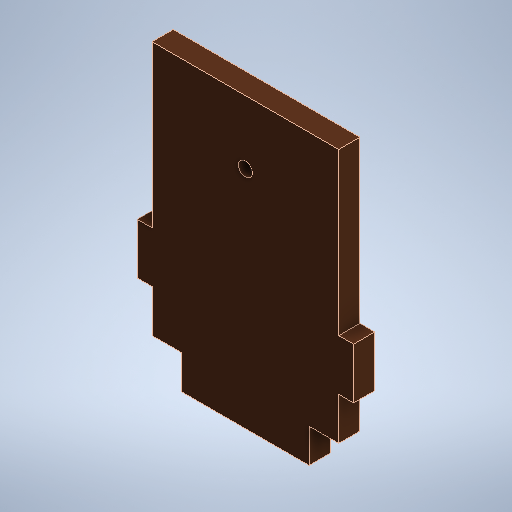
# Autodesk Inventor part: Path Back End
Saved by Autodesk Inventor 2025.4 (Build 294407000, 407)
## iProperties
Created: 2026-04-10
Part Number: Path Back End
Material: Generic
Document SubType Name: Sheet Metal
Designer: lenovo
Density: 1 g/cm^3
Sheet Metal Rule: Default_mm
Appearance: Default(1)
Author: lenovo
Autodesk Inventor part; units mm, degrees
ref_plane "YZ Plane" through (0, 0, 0) normal (1, 0, 0) x (0, 1, 0)
ref_plane "XZ Plane" through (0, 0, 0) normal (0, 1, 0) x (-1, 0, 0)
ref_plane "XY Plane" through (0, 0, 0) normal (0, 0, 1) x (1, 0, 0)
sketch "Sketch1" plane through (0, 0, 0) normal (0, 0, 1) x (1, 0, 0)
  line L0 (-22, -30) -> (22, -30)
  line L1 (22, -30) -> (22, 30)
  line L2 (22, 30) -> (-22, 30)
  line L3 (-22, 30) -> (-22, -30)
  line L4 (-22, -30) -> (22, 30) construction
  line L5 (22, -30) -> (-22, 30) construction
  line L6 (-15, -38) -> (15, -38)
  line L7 (15, -38) -> (15, -30)
  line L8 (15, -30) -> (-15, -30)
  line L9 (-15, -30) -> (-15, -38)
  line L10 (-15, -38) -> (15, -30) construction
  line L11 (15, -38) -> (-15, -30) construction
  circle A0 centre (0, 15) radius 1.65
  point P0 (0, 0)
  point P1 (0, -34)
  point P2 (0, -30)
  point P3 (0, 30)
  dimension "d0" = 44
  dimension "d1" = 60
  dimension "d2" = 30
  dimension "d3" = 8
  dimension "d4" = 3.3
  dimension "d5" = 15
  measures "d0" distance of L1.end L2.end
  measures "d1" distance of L0.end L1.end
  measures "d2" distance of L6.start L6.end
  measures "d3" distance of L6.end L7.end
  measures "d4" diameter of A0
  measures "d5" distance from line of L2 A0.centre
sketch "Sketch2" plane through (0, 0, 5) normal (0, 0, 1) x (1, 0, 0)
  line L0 (22, -30) -> (22, 30)
  line L1 (22, -20) -> (25.5, -20)
  line L2 (25.5, -20) -> (25.5, -8)
  line L3 (25.5, -8) -> (22, -8)
  line L4 (22, -8) -> (22, -20)
  line L5 (22, -30) -> (15, -30)
  line L6 (0, 0) -> (0, -38)
  line L7 (-15, -38) -> (15, -38)
  line L8 (-22, -20) -> (-25.5, -20)
  line L9 (-25.5, -20) -> (-25.5, -8)
  line L10 (-25.5, -8) -> (-22, -8)
  line L11 (-22, -8) -> (-22, -20)
  dimension "d7" = 3.5
  dimension "d8" = 12
  dimension "d9" = 10
  measures "d7" distance of L2.end L3.end
  measures "d8" distance of L1.end L2.end
  measures "d9" distance between parallel lines of L5 L1
extrude "Plate1" add sketch "Sketch1" along normal blind 5
sheet face with bend "Face2" sketch "Sketch2" thickness 5 toward (0, 0, -1) bend radius 5
bend "Bend1"
equation "\"d6\" = Thickness"
equation "\"d10\" = BendRadius"
equation "\"d11\" = BendReliefWidth"
equation "\"d13\" = MinimumRemnant"
equation "\"d12\" = BendReliefDepth"
equation "\"d14\" = TransitionRadius"
equation "\"BendRadius\" = Thickness"
equation "\"BendReliefWidth\" = Thickness"
equation "\"BendReliefDepth\" = 0.5 * Thickness"
equation "\"TransitionRadius\" = BendRadius"
equation "\"JacobiRadiusSize\" = BendRadius"
equation "\"GapSize\" = Thickness"
equation "\"Thickness\" = 5"
equation "\"MinimumRemnant\" = 10"
body "Solid1"
